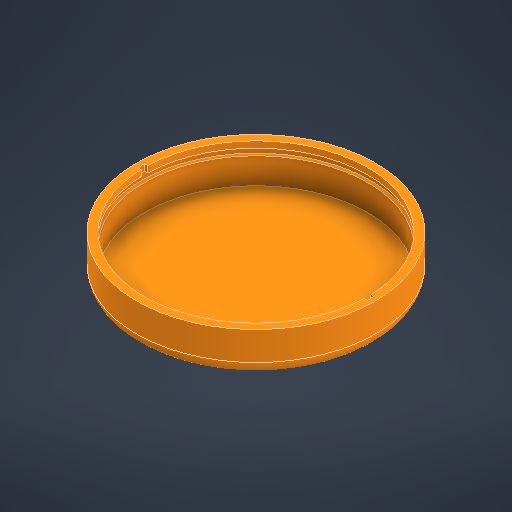
# Autodesk Inventor part: Poklop
Saved by Autodesk Inventor 2026.1 (Build 301233000, 233)
## iProperties
Created: 2025-10-01
Part Number: Poklop
Material: Všeobecné
Document SubType Name: Modeling
Designer: cerna
Density: 1 g/cm^3
Appearance: Oranžová
Author: cerna
Autodesk Inventor part; units mm, degrees
ref_plane "YZ Plane" through (0, 0, 0) normal (1, 0, 0) x (0, 1, 0)
ref_plane "XZ Plane" through (0, 0, 0) normal (0, 1, 0) x (-1, 0, 0)
sketch "Náčrt1" plane through (0, 0, 0) normal (0, 1, 0) x (-1, 0, 0)
  circle A0 centre (0, 0) radius 92
  dimension "d0" = 184
  constraints: 1 centre point, 1 coincident
  measures "d0" diameter of A0
extrude "Vysunutí1" add sketch "Náčrt1" along normal blind 2
sketch "Náčrt2" plane through (0, 2, 0) normal (0, 1, 0) x (1, 0, 0)
  circle A0 centre (0, 0) radius 86
  circle A1 centre (0, 0) radius 92
  dimension "d3" = 184
  dimension "d8" = 172
  constraints: 2 centre point, 2 coincident
  measures "d3" diameter of A1
  measures "d8" diameter of A0
extrude "Vysunutí2" add sketch "Náčrt2" along normal blind 30
ref_plane "Pracovní rovina1" through (0, 22, 0) normal (0, 1, 0) x (1, 0, 0)
sketch "Náčrt3" plane through (0, 22, 0) normal (0, 1, 0) x (1, 0, 0)
  circle A0 centre (0, 0) radius 88.5
  dimension "d7" = 177
  constraints: 1 centre point, 1 coincident
  measures "d7" diameter of A0
extrude "Vysunutí3" cut sketch "Náčrt3" along normal blind 5.1
sketch "Náčrt4" plane through (0, 32, 0) normal (0, 1, 0) x (1, 0, 0)
  circle A0 centre (0, 0) radius 88.5 projected
  line L0 (-88.4633, 2.55) -> (-84.4633, 2.55)
  line L1 (-84.4633, 2.55) -> (-84.4633, -2.55)
  line L2 (-84.4633, -2.55) -> (-88.4633, -2.55)
  line L3 (-88.4633, -2.55) -> (-88.4633, 2.55)
  line L4 (0, 128.8) -> (0, -128.8) projected
  line L5 (128.8, 0) -> (-128.8, 0) projected
  line L6 (84.4633, 2.55) -> (88.4633, 2.55)
  line L7 (88.4633, 2.55) -> (88.4633, -2.55)
  line L8 (88.4633, -2.55) -> (84.4633, -2.55)
  line L9 (84.4633, -2.55) -> (84.4633, 2.55)
  dimension "d11" = 4
  dimension "d12" = 5.1
  dimension "d15" = 360
  constraints: 16 end point, 3 parallel, 1 horizontal, 1 perpendicular, 20 other
  measures "d11" distance of L1.end L2.end
  measures "d12" distance of L0.end L1.end
extrude "Vysunutí4" cut sketch "Náčrt4" against normal blind 5.1 contours L7 L5 L9 L6 | L8 L9 L5 L7 | L0 L1 L5 L3 | L3 L5 L1 L2
fillet "Zaoblení1" radius 10 1 edges at (92, 0, 0)
